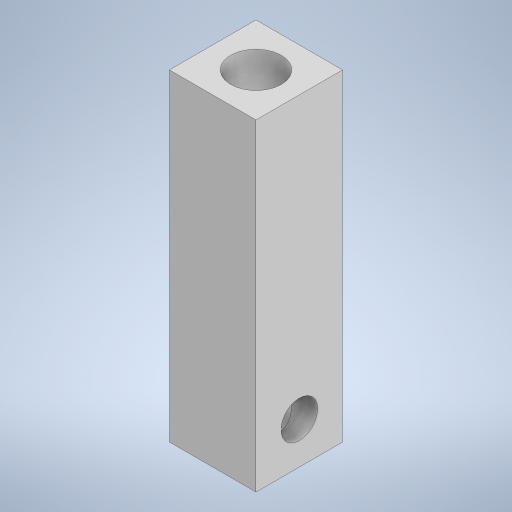
# Autodesk Inventor part: wheel-lock
Saved by Autodesk Inventor 2024.2 (Build 282272000, 272)
## iProperties
Created: 2024-04-01
Part Number: wheel-lock
Material: Generic
Document SubType Name: Modeling
Designer: Robin
Density: 1 g/cm^3
Appearance: Default
Author: Robin
Autodesk Inventor part; units mm, degrees
ref_plane "YZ Plane" through (0, 0, 0) normal (1, 0, 0) x (0, 1, 0)
ref_plane "XZ Plane" through (0, 0, 0) normal (0, 1, 0) x (-1, 0, 0)
ref_plane "XY Plane" through (0, 0, 0) normal (0, 0, 1) x (1, 0, 0)
sketch "Sketch1" plane through (0, 0, 0) normal (0, 1, 0) x (-1, 0, 0)
  line L0 (4.7, 4.7) -> (-4.7, 4.7)
  line L1 (-4.7, 4.7) -> (-4.7, -4.7)
  line L2 (-4.7, -4.7) -> (4.7, -4.7)
  line L3 (4.7, -4.7) -> (4.7, 4.7)
  point P0 (0, 0)
  point P1 (4.7, 0)
  point P2 (0, -4.7)
  dimension "d0" = 9.4
  dimension "d1" = 9.4
  constraints: 8 end point, 2 midpoint, 2 parallel, 1 horizontal, 1 horizontal alignment, 1 perpendicular, 1 vertical alignment
  measures "d0" distance of L2.end L0.start
  measures "d1" distance of L1.end L2.end
extrude "Extrusion1" add sketch "Sketch1" along normal blind 35
sketch "Sketch2" plane through (0, 35, 0) normal (0, 1, 0) x (1, 0, 0)
  circle A0 centre (0, 0) radius 2.75
  dimension "d4" = 5.5
  constraints: 1 centre point, 1 coincident
  measures "d4" diameter of A0
extrude "Extrusion2" cut sketch "Sketch2" against normal through all
sketch "Sketch3" plane through (4.7, 0, 4.7) normal (1, 0, 0) x (0, 0, -1)
  circle A0 centre (4.7, 4.5) radius 2
  line L0 (0, 0) -> (9.4, 0) projected
  point P0 (4.7, 0)
  point P1 (4.7, 0)
  point P2 (4.7, 0)
  dimension "d7" = 4
  dimension "d8" = 4.5
  constraints: 2 midpoint, 1 centre point, 1 vertical alignment
  measures "d7" diameter of A0
  measures "d8" distance of point (4.7, 0) A0.centre
extrude "Extrusion3" cut sketch "Sketch3" against normal blind 5
body "Solid1"
